Bag Cap July 13 (Autodesk Fusion 360 design; units mm, degrees)
Autodesk Fusion 360 part; units mm, degrees
note: some values were not read from the file. Set by a fixed rule: which sketch regions a step uses.
sketch "Sketch1" plane through (0, 0, 0) normal (0, 0, 1) x (1, 0, 0)
  circle A0 centre (0, 0) radius 10.414
  circle A1 centre (0, 0) radius 12.319
  dimension "d1" = 20.828
  dimension "d2" = 1.905
  measures "d1" diameter of A0
extrude "Extrude1" add sketch "Sketch1" along normal blind 12.7 makes body 1
sketch "Sketch2" plane through (0, 0, 12.7) normal (0, 0, 1) x (1, 0, 0)
  circle A0 centre (0, 0) radius 10.414
  circle A1 centre (0, 0) radius 12.319
  circle A2 centre (0, 0) radius 7.62
  dimension "d5" = 15.24
  measures "d5" diameter of A2
extrude "Extrude2" add sketch "Sketch2" along normal blind 3.175 contours A0 | A1 bodies 1
sketch "Sketch3" plane through (0, 0, 0) normal (0, 0, -1) x (-1, 0, 0)
  circle A0 centre (0, 0) radius 10.414
  circle A1 centre (0, 0) radius 12.319
  circle A2 centre (0, 0) radius 10.414
coil "CoilPrimitive1" add diameter 21.082 section circle size 2.032 on centre turns 3 pitch 2.54 right hand placed x (-1, 0, 0) y (0, -1, 0) z (0, 0, 1) at (0, 0, 0) bodies 1
extrude "Extrude3" cut sketch "Sketch3" along normal blind 2.54 contours A0 A2 | A1 bodies 1
sketch "Sketch5" plane through (0, 0, 15.875) normal (0, 0, 1) x (1, 0, 0)
  circle A0 centre (0, 0) radius 7.62
  circle A1 centre (0, 0) radius 12.319
  line L0 (-2.54, 13.97) -> (2.54, 13.97)
  line L1 (2.54, 13.97) -> (2.54, -13.97)
  line L2 (2.54, -13.97) -> (-2.54, -13.97)
  line L3 (-2.54, -13.97) -> (-2.54, 13.97)
  line L4 (13.97, -2.54) -> (-13.97, -2.54)
  line L5 (-13.97, -2.54) -> (-13.97, 2.54)
  line L6 (13.97, 2.54) -> (13.97, -2.54)
  line L7 (-13.97, 2.54) -> (13.97, 2.54)
  line L8 (2.54, 13.97) -> (2.54, -13.97)
  line L9 (2.54, -13.97) -> (-2.54, -13.97)
  line L10 (-2.54, 13.97) -> (2.54, 13.97)
  line L11 (-2.54, -13.97) -> (-2.54, 13.97)
  line L12 (-13.97, 2.54) -> (13.97, 2.54)
  line L13 (13.97, 2.54) -> (13.97, -2.54)
  line L14 (-13.97, -2.54) -> (-13.97, 2.54)
  line L15 (13.97, -2.54) -> (-13.97, -2.54)
  circle A2 centre (-43.7185, -43.7185) radius 50.8
  circle A3 centre (43.7185, -43.7185) radius 50.8
  circle A4 centre (43.7185, 43.7185) radius 50.8
  circle A5 centre (-43.7185, 43.7185) radius 50.8
  circle A6 centre (0, 0) radius 12.319
  point P0 (2.54, 0)
  point P1 (0, -13.97)
  dimension "d15" = 27.94
  dimension "d16" = 5.08
  dimension "d18" = 360
  dimension "d19" = 101.6
  dimension "d21" = 360
  measures "d15" distance of L0.end L1.end
  measures "d16" distance of L0.start L0.end
  measures "d19" diameter of A2
extrude "Extrude4" add sketch "Sketch5" against normal up to surface (15.875 mm away) contours A1 L4 L6 L7 L12 L13 L15 A6 | A1 L7 L12 A4 A6 | A1 L4 L15 A3 A6 | A1 L1 L8 A4 A6 | A1 L0 L1 L3 L8 L10 L11 A6 | A1 L1 L2 L3 L8 L9 L11 A6 | A1 L1 L8 A3 A6 | A1 L3 L11 A5 A6 | A1 L3 L11 A2 A6 | A1 L7 L12 A5 A6 | A1 L4 L5 L7 L12 L14 L15 A6 | A1 L4 L15 A2 A6 bodies 1
chamfer "Chamfer1" distance 1.27 angle 45 1 edges at (-7.1043, 2.7555, 15.875) on bodies 1
chamfer "Chamfer2" distance 1.27 angle 45 1 edges at (-7.1043, 2.7555, 12.7) on bodies 1
sketch "Sketch6" plane through (0, 0, 0) normal (1, 0, 0) x (0, 0, -1)
  line L0 (-13.97, 7.62) -> (-13.97, -7.62) construction
  line L1 (-12.7, -8.89) -> (-12.7, 8.89) construction
  line L2 (-11.3684, -9.144) -> (-15.24, -5.2724)
  line L3 (0, 4.4543) -> (-15.875, 4.4543)
  line L4 (-15.24, -5.2724) -> (-15.24, -1.016)
  line L5 (-15.24, -1.016) -> (-11.3684, -1.016)
  line L6 (-13.97, -7.62) -> (-12.7, -8.89) construction
  line L7 (-15.875, 0) -> (-12.7, 0) construction
  line L8 (-15.24, -2.3812) -> (-25.4, -2.3812)
  line L9 (-11.3684, -9.144) -> (-11.3684, -1.016)
  line L10 (-15.24, -1.016) -> (-25.4, -1.016)
  line L11 (-25.4, -1.016) -> (-25.4, -2.3812)
  line L12 (-25.4, -2.3812) -> (-19.05, -3.3972)
  line L13 (-19.05, -3.3972) -> (-19.05, -2.3812)
  line L14 (-11.3684, -7.3152) -> (-6.2884, -7.3152)
  line L15 (-15.875, -4.4543) -> (0, -4.4543)
  line L16 (-6.2884, -7.3152) -> (-6.2884, -1.016)
  line L17 (-6.2884, -1.016) -> (-11.3684, -1.016)
  line L18 (-11.6224, -8.89) -> (-11.6224, -9.144)
  line L19 (-11.6224, -9.144) -> (-11.3684, -9.144)
  line L20 (-11.3684, -9.144) -> (-10.0984, -9.144)
  line L21 (-10.0984, -9.144) -> (-10.0984, -7.3152)
  point P0 (-15.875, 0)
  point P1 (-12.7, 0)
  dimension "d26" = 0.762
  dimension "d27" = 1.27
  dimension "d28" = 1.016
  dimension "d29" = 2.3813
  dimension "d30" = 10.16
  dimension "d31" = 0.254
  dimension "d32" = 1.016
  dimension "d33" = 6.35
  dimension "d37" = 5.08
  dimension "d38" = 7.3152
  dimension "d40" = 1.27
  measures "d26" distance of L0.end L2
  measures "d27" distance of L0.end L2.end
  measures "d28" distance of L5 L7
  measures "d29" distance of L7 L8
  measures "d30" distance of L8.start L8.end
  measures "d31" distance of L2.start L1.start
  measures "d32" distance of L12.end L13.end
  measures "d33" distance of L8.end L13.end
  measures "d37" distance of L14.start L14.end
  measures "d38" distance of P1 L14.end
  measures "d40" distance of L9 L21
revolve "Revolve1" add sketch "Sketch6" angle 360 about axis through (0, 0, 15.875) along (0, 0, -1) separate body contours L2 L4 L9 L15 | L9 L14 L20 L21 | L9 L14 L15 L16 | L4 L5 L9 L15 | L9 L15 L16 L17 | L4 L8 L10 L11 | L8 L12 L13 makes body 2
fillet "Fillet1" radius 7.112 1 edges at (-4.9156, -1.9066, 15.24) on bodies 2
sketch "Sketch10" plane through (0, 0, 15.875) normal (0, 0, 1) x (1, 0, 0)
  arc A0 (4.4543, -11.4855) -> (11.4855, -4.4543) centre (0, 0) ccw
  arc A1 (13.97, -2.54) -> (11.4855, -4.4543) centre (43.7185, -43.7185) ccw
  line L0 (13.97, -2.54) -> (13.97, 2.54)
  arc A2 (11.4855, 4.4543) -> (13.97, 2.54) centre (43.7185, 43.7185) ccw
  arc A3 (11.4855, 4.4543) -> (4.4543, 11.4855) centre (0, 0) ccw
  arc A4 (2.54, 13.97) -> (4.4543, 11.4855) centre (43.7185, 43.7185) ccw
  line L1 (2.54, 13.97) -> (-2.54, 13.97)
  arc A5 (-4.4543, 11.4855) -> (-2.54, 13.97) centre (-43.7185, 43.7185) ccw
  arc A6 (-4.4543, 11.4855) -> (-11.4855, 4.4543) centre (0, 0) ccw
  arc A7 (-13.97, 2.54) -> (-11.4855, 4.4543) centre (-43.7185, 43.7185) ccw
  line L2 (-13.97, 2.54) -> (-13.97, -2.54)
  arc A8 (-11.4855, -4.4543) -> (-13.97, -2.54) centre (-43.7185, -43.7185) ccw
  arc A9 (-11.4855, -4.4543) -> (-4.4543, -11.4855) centre (0, 0) ccw
  arc A10 (-2.54, -13.97) -> (-4.4543, -11.4855) centre (-43.7185, -43.7185) ccw
  line L3 (-2.54, -13.97) -> (2.54, -13.97)
  arc A11 (4.4543, -11.4855) -> (2.54, -13.97) centre (43.7185, -43.7185) ccw
  circle A12 centre (0, 0) radius 8.89
  line L4 (-13.97, 2.54) -> (-2.54, 2.54)
  line L5 (-2.54, 2.54) -> (-2.54, -13.97)
  line L6 (-2.54, -13.97) -> (-8.97, -13.97)
  line L7 (-13.97, -13.97) -> (-13.97, 2.54)
  arc A13 (-11.4855, -4.4543) -> (-4.4543, -11.4855) centre (0, 0) ccw
  arc A14 (-11.4855, -4.4543) -> (-13.97, -2.54) centre (-43.7185, -43.7185) ccw
  arc A15 (-2.54, -13.97) -> (-4.4543, -11.4855) centre (-43.7185, -43.7185) ccw
  line L8 (-13.97, -13.97) -> (-13.97, -23.97)
  line L9 (-13.97, -23.97) -> (-8.97, -23.97)
  line L10 (-8.97, -23.97) -> (-8.97, -13.97)
  dimension "d43" = 10
  dimension "d44" = 5
  measures "d43" distance of A10.start L9
  measures "d44" distance of L8 L10
extrude "Extrude5" add sketch "Sketch10" against normal up to surface (15.875 mm away) contours A8 A9 A10 L6 L7 A13 A14 A15 L8 L9 L10 bodies 1
fillet "Fillet2" radius 2 1 edges at (-8.97, -13.97, 7.9375) on bodies 1
sketch "Sketch12" plane through (0, -23.97, 0) normal (0, -1, 0) x (1, 0, 0)
  line L0 (-13.97, 0) -> (-8.97, 0)
  line L1 (-8.97, 0) -> (-8.97, 15.875)
  line L2 (-8.97, 15.875) -> (-13.97, 15.875)
  line L3 (-13.97, 15.875) -> (-13.97, 0)
  line L4 (-13.97, 9.4875) -> (-15.97, 9.4875)
  line L5 (-15.97, 9.4875) -> (-15.97, 6.3875)
  line L6 (-15.97, 6.3875) -> (-13.97, 6.3875)
  line L7 (-13.97, 6.3875) -> (-13.97, 9.4875)
  line L8 (-15.97, 10.5875) -> (-19.27, 10.5875)
  line L9 (-19.27, 10.5875) -> (-19.27, 5.2875)
  line L10 (-19.27, 5.2875) -> (-15.97, 5.2875)
  line L11 (-15.97, 5.2875) -> (-15.97, 10.5875)
  point P0 (-13.97, 7.9375)
  point P1 (-15.97, 7.9375)
  dimension "d51" = 3.1
  dimension "d52" = 2
  dimension "d53" = 5.3
  dimension "d54" = 3.3
  measures "d51" distance of L4.end L5.end
  measures "d52" distance of L5.end L6.end
  measures "d53" distance of L8.end L9.end
  measures "d54" distance of L8.start L8.end
extrude "Extrude7" add sketch "Sketch12" against normal blind 26.51 contours L3 L4 L5 L6 L7 L11 | L5 L8 L9 L10 L11 bodies 1
fillet "Fillet3" radius 1.5 2 edges at (-13.97, -10.715, 9.4875) (-13.97, -10.715, 6.3875) on bodies 1
chamfer "Chamfer3" distance 1 angle 45 1 edges at (-6.8202, -2.6453, 6.2884) on bodies 2
chamfer "Chamfer4" distance 0.5 angle 45 1 edges at (-6.8202, -2.6453, 10.0984) on bodies 2
chamfer "Chamfer5" distance 1.2 angle 45 2 edges at (-19.27, -10.715, 10.5875) (-19.27, -10.715, 5.2875) on bodies 1
equation "d29 = 3 / 16 * 0.5 in"
